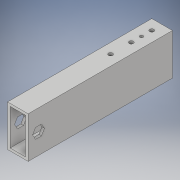
# Autodesk Inventor part: 1X2 7in
Saved by Autodesk Inventor 2018 (Build 220112000, 112)
## iProperties
Created: 2019-01-11
Part Number: 1X2 7in
Material: Generic
Document SubType Name: Modeling
Designer: s-2512711
Density: 1 g/cm^3
Appearance: Default
Author: s-2512711
Autodesk Inventor part; units mm, degrees
ref_plane "YZ Plane" through (0, 0, 0) normal (1, 0, 0) x (0, 1, 0)
ref_plane "XZ Plane" through (0, 0, 0) normal (0, 1, 0) x (-1, 0, 0)
ref_plane "XY Plane" through (0, 0, 0) normal (0, 0, 1) x (1, 0, 0)
sketch "Sketch1" plane through (0, 0, 0) normal (0, 0, 1) x (1, 0, 0)
  line L0 (0, 0) -> (25.4, 0)
  line L1 (25.4, 0) -> (25.4, 50.8)
  line L2 (25.4, 50.8) -> (0, 50.8)
  line L3 (0, 50.8) -> (0, 0)
  line L4 (3.175, 47.625) -> (22.225, 47.625)
  line L5 (22.225, 47.625) -> (22.225, 3.175)
  line L6 (22.225, 3.175) -> (3.175, 3.175)
  line L7 (3.175, 3.175) -> (3.175, 47.625)
  dimension "d0" = 25.4
  dimension "d1" = 50.8
  dimension "d2" = 3.175
  constraints: 16 end point, 4 parallel, 2 perpendicular, 1 horizontal, 3 other
  measures "d0" distance of L2.end L1.end
  measures "d1" distance of L1.end L0.end
  measures "d2" distance between parallel lines of L2 L4
extrude "Extrusion1" add sketch "Sketch1" along normal blind 177.8
sketch "Sketch2" plane through (25.4, 0, 0) normal (1, 0, 0) x (0, 0, -1)
  line L0 (-177.8, 47.625) -> (-177.8, 3.175) projected
  line L1 (-177.8, 25.4) -> (-165.1, 25.4) construction
  line L2 (-172.4323, 25.4) -> (-168.7662, 31.75)
  line L3 (-168.7662, 31.75) -> (-161.4338, 31.75)
  line L4 (-161.4338, 31.75) -> (-157.7677, 25.4)
  line L5 (-157.7677, 25.4) -> (-161.4338, 19.05)
  line L6 (-161.4338, 19.05) -> (-168.7662, 19.05)
  line L7 (-168.7662, 19.05) -> (-172.4323, 25.4)
  point P0 (0, 0)
  dimension "d5" = 12.7
  dimension "d6" = 12.7
  constraints: 14 end point, 1 coincident, 1 horizontal, 1 midpoint, 13 other
  measures "d5" distance of L1.start L1.end
  measures "d6" distance between parallel lines of L6 L3
extrude "Extrusion2" cut sketch "Sketch2" against normal blind 177.8
sketch "Sketch3" plane through (0, 50.8, 0) normal (0, 1, 0) x (1, 0, 0)
  line L0 (25.4, 0) -> (0, 0) projected
  line L1 (12.7, 0) -> (12.7, -25.4) construction
  line L2 (12.7, 0) -> (38.1, 0) construction
  circle A0 centre (12.7, -25.4) radius 1.9844
  dimension "d9" = 25.4
  dimension "d10" = 90
  dimension "d11" = 3.9688
  constraints: 4 end point, 1 centre point, 1 coincident, 1 horizontal, 1 midpoint, 1 perpendicular, 1 vertical
  measures "d9" distance of L1.start L1.end
  measures "d10" angle of L1 L2
  measures "d11" diameter of A0
extrude "Extrusion3" cut sketch "Sketch3" against normal blind 76.2
sketch "Sketch4" plane through (0, 50.8, 0) normal (0, 1, 0) x (1, 0, 0)
  line L0 (3.175, 0) -> (22.225, 0) construction
  line L1 (12.7, 0) -> (12.7, -12.7) construction
  line L2 (12.7, -12.7) -> (12.7, -38.1) construction
  line L3 (12.7, -38.1) -> (12.7, -63.5) construction
  circle A0 centre (12.7, -12.7) radius 2.5797
  circle A1 centre (12.7, -38.1) radius 2.5797
  circle A2 centre (12.7, -63.5) radius 2.5797
  point P0 (0, 0)
  dimension "d14" = 12.7
  dimension "d15" = 25.4
  dimension "d16" = 25.4
  dimension "d17" = 5.1594
  constraints: 6 end point, 3 centre point, 3 coincident, 2 point on line, 1 midpoint, 1 vertical
  measures "d14" distance of L1.start L1.end
  measures "d15" distance of L1.end L2.end
  measures "d16" distance of L2.end L3.end
  measures "d17" diameter of A0
extrude "Extrusion4" cut sketch "Sketch4" against normal blind 68.2625
body "Solid1"
